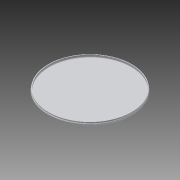
# Autodesk Inventor part: Disceep20CaseBottom
Saved by Autodesk Inventor 2014 (Build 180170000, 170)
## iProperties
Created: 2014-11-30
Part Number: Disceep20CaseBottom
Material: Generic
Document SubType Name: Modeling
Designer: DV
Density: 1 g/cm^3
Appearance: Default
Author: DV
Autodesk Inventor part; units mm, degrees
ref_plane "YZ Plane" through (0, 0, 0) normal (1, 0, 0) x (0, 1, 0)
ref_plane "XZ Plane" through (0, 0, 0) normal (0, 1, 0) x (-1, 0, 0)
ref_plane "XY Plane" through (0, 0, 0) normal (0, 0, 1) x (1, 0, 0)
sketch "Sketch1" plane through (0, 0, 0) normal (0, 0, 1) x (1, 0, 0)
  line L0 (-3.4203, -12.5273) -> (3.4203, -12.5273)
  line L1 (3.4203, -12.5273) -> (5.8707, -13.3236)
  arc A0 (6.1763, -13.6922) -> (5.8707, -13.3236) centre (5.7324, -13.7494) ccw
  arc A1 (6.1763, -13.6922) -> (7.2484, -14.6351) centre (7.2484, -13.5542) ccw
  line L2 (7.2484, -14.6351) -> (7.758, -14.6351)
  arc A2 (8.4318, -15.3089) -> (7.758, -14.6351) centre (7.758, -15.3089) ccw
  line L3 (8.4318, -15.3089) -> (8.4318, -18.2648)
  arc A3 (8.254, -18.384) -> (8.4318, -18.2648) centre (8.3829, -18.384) ccw
  line L4 (8.254, -18.384) -> (8.254, -15.3089)
  arc A4 (8.254, -15.3089) -> (7.758, -14.8129) centre (7.758, -15.3089) ccw
  line L5 (7.758, -14.8129) -> (7.2484, -14.8129)
  arc A5 (6, -13.7149) -> (7.2484, -14.8129) centre (7.2484, -13.5542) ccw
  arc A6 (6, -13.7149) -> (5.8158, -13.4927) centre (5.7324, -13.7494) ccw
  line L6 (5.8158, -13.4927) -> (3.3921, -12.7051)
  line L7 (3.3921, -12.7051) -> (-3.3921, -12.7051)
  line L8 (-3.3921, -12.7051) -> (-5.8158, -13.4927)
  arc A7 (-5.8158, -13.4927) -> (-6, -13.7149) centre (-5.7324, -13.7494) ccw
  arc A8 (-7.2484, -14.8129) -> (-6, -13.7149) centre (-7.2484, -13.5542) ccw
  line L9 (-7.2484, -14.8129) -> (-7.758, -14.8129)
  arc A9 (-7.758, -14.8129) -> (-8.254, -15.3089) centre (-7.758, -15.3089) ccw
  line L10 (-8.254, -15.3089) -> (-8.254, -18.384)
  arc A10 (-8.4318, -18.2648) -> (-8.254, -18.384) centre (-8.3829, -18.384) ccw
  line L11 (-8.4318, -18.2648) -> (-8.4318, -15.3089)
  arc A11 (-7.758, -14.6351) -> (-8.4318, -15.3089) centre (-7.758, -15.3089) ccw
  line L12 (-7.758, -14.6351) -> (-7.2484, -14.6351)
  arc A12 (-7.2484, -14.6351) -> (-6.1763, -13.6922) centre (-7.2484, -13.5542) ccw
  arc A13 (-5.8707, -13.3236) -> (-6.1763, -13.6922) centre (-5.7324, -13.7494) ccw
  line L13 (-5.8707, -13.3236) -> (-3.4203, -12.5273)
  line L14 (-8.4318, -17.9755) -> (-8.5588, -17.9755)
  line L15 (-8.5588, -17.9755) -> (-8.5588, -18.1882)
  line L16 (0, -9.0987) -> (0, -22.0894) construction
  line L17 (-8.3829, -18.5129) -> (0, -18.5129)
  line L18 (0, -18.5129) -> (0, -18.6472)
  line L19 (0, -18.6472) -> (-8.3829, -18.6472)
  arc A14 (-8.5588, -18.1882) -> (-8.3829, -18.6472) centre (-8.3829, -18.384) ccw
  point P0 (0, 0)
  dimension "d0" = 0.127
  constraints: 40 end point, 31 point on circle, 15 centre point, 7 horizontal, 4 vertical, 3 perpendicular, 2 parallel, 2 point on line, 1 coincident, 1 tangent, 60 other
  measures "d0" distance of L14.start L14.end
revolve "Revolution1" add sketch "Sketch1" angle 360 about axis through (0, -9.0987, 0) along (0, -1, 0) contours L11 A10 L17 L18 L19 A14 L15 L14
body "Solid1"
